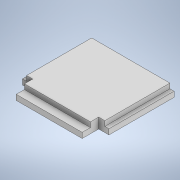
# Autodesk Inventor part: External interface bottom
Saved by Autodesk Inventor 2020 (Build 240168000, 168)
## iProperties
Created: 2019-06-27
Part Number: External interface bottom
Material: Generic
Document SubType Name: Modeling
Designer: cruss
Density: 1 g/cm^3
Appearance: Default
Author: cruss
## iProperties of the stored document _3DPrint.ipt
Created: 2019-07-11
Part Number: _3DPrint
Material: Generic
Document SubType Name: Modeling
Designer: cruss
Density: 1 g/cm^3
Appearance: Default
Author: cruss
Autodesk Inventor part; units mm, degrees
ref_plane "YZ Plane" through (0, 0, 0) normal (1, 0, 0) x (0, 1, 0)
ref_plane "XZ Plane" through (0, 0, 0) normal (0, 1, 0) x (-1, 0, 0)
ref_plane "XY Plane" through (0, 0, 0) normal (0, 0, 1) x (1, 0, 0)
sketch "Sketch4" plane through (0, 0, 0) normal (0, 1, 0) x (-1, 0, 0)
  line L0 (0, 0) -> (26.67, 0)
  line L1 (26.67, 0) -> (26.67, 20.066)
  line L2 (26.67, 20.066) -> (0, 20.066)
  line L3 (0, 20.066) -> (0, 0)
  dimension "d20" = 20.066
  dimension "d21" = 26.67
  constraints: 8 end point, 2 parallel, 1 horizontal, 1 perpendicular
  measures "d20" distance of L0.end L1.end
  measures "d21" distance of L1.end L2.end
extrude "Extrusion4" add sketch "Sketch4" along normal blind 1.651
sketch "Sketch5" plane through (0, 1.651, 0) normal (0, 1, 0) x (1, 0, 0)
  line L0 (-26.67, -20.066) -> (0, -20.066) projected
  line L1 (-25.4, -20.066) -> (-1.27, -20.066)
  line L2 (-1.27, -20.066) -> (-1.27, 0)
  line L3 (-1.27, 0) -> (-25.4, 0)
  line L4 (-25.4, 0) -> (-25.4, -20.066)
  line L5 (-26.67, 0) -> (-26.67, -20.066) projected
  line L6 (0, 0) -> (-26.67, 0) projected
  line L7 (0, -20.066) -> (0, 0) projected
  point P0 (-1.27, -20.066)
  dimension "d24" = 1.27
  dimension "d25" = 0
  dimension "d26" = 1.27
  constraints: 8 end point, 2 parallel, 1 horizontal, 1 perpendicular, 1 point on line
  measures "d24" distance between parallel lines of L5 L4
  measures "d25" distance between parallel lines of L6 L3
  measures "d26" distance between parallel lines of L7 L2
extrude "Extrusion5" add sketch "Sketch5" along normal blind 1.524 contours L4 L3 L2 L0
sketch "Sketch8" plane through (-26.67, 0, 20.066) normal (0, 0, 1) x (1, 0, 0)
  line L0 (3.175, 1.651) -> (23.495, 1.651)
  line L1 (23.495, 1.651) -> (23.495, 0)
  line L2 (23.495, 0) -> (3.175, 0)
  line L3 (3.175, 0) -> (3.175, 1.651)
  line L4 (0, 0) -> (26.67, 0) projected
  line L5 (26.67, 0) -> (26.67, 1.651) projected
  line L6 (0, 0) -> (0, 1.651) projected
  dimension "d42" = 20.32
  dimension "d43" = 1.651
  dimension "d44" = 0
  dimension "d45" = 26.67
  dimension "d46" = 3.175
  constraints: 8 end point, 2 parallel, 1 horizontal, 1 perpendicular
  measures "d42" distance of L0.start L0.end
  measures "d43" distance of L0.end L1.end
  measures "d44" distance between parallel lines of L4 L2
  measures "d45" distance between parallel lines of L5 L6
  measures "d46" distance between parallel lines of L3 L6
extrude "Extrusion8" add sketch "Sketch8" along normal blind 5.08
sketch "Sketch9" plane through (-23.495, 1.651, 20.066) normal (0, 1, 0) x (1, 0, 0)
  line L0 (0, 0) -> (0, -5.08) projected
  line L1 (20.32, -2.54) -> (0, -2.54)
  line L2 (0, 0) -> (20.32, 0)
  line L3 (20.32, 0) -> (20.32, -2.54)
  line L4 (20.32, -2.54) -> (0, -2.54)
  line L5 (0, -2.54) -> (0, 0)
  point P0 (23.495, 20.066)
  constraints: 10 end point, 2 parallel, 1 horizontal, 1 perpendicular
extrude "Extrusion9" add sketch "Sketch9" along normal blind 1.524
equation "\"d26\" = d24"
equation "\"d46\" = -0.5 * d42 + 0.5 * d45"
body "Solid2"
